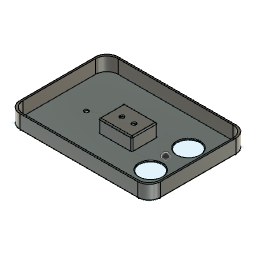
topo novo (Autodesk Fusion 360 design; units mm, degrees)
Autodesk Fusion 360 part; units mm, degrees
note: some values were not read from the file. Chosen so that the rebuilt part matches the saved one: which pieces of a blend or face edit are solid.
sketch "Esboço1" plane through (0, 0, 0) normal (0, 0, 1) x (1, 0, 0)
  line L0 (93, 65) -> (-93, 65)
  line L1 (-93, 65) -> (-93, -65)
  line L2 (-93, -65) -> (93, -65)
  line L3 (93, -65) -> (93, 65)
  line L4 (93, 65) -> (-93, -65) construction
  line L5 (-93, 65) -> (93, -65) construction
  dimension "d1" = 186
  dimension "d2" = 130
  constraint horizontal L0
  constraint perpendicular L0 L1
  constraint parallel L0 L2
  constraint parallel L1 L3
  constraint coincident L4 origin
  constraint coincident L5 origin
  measures "d1" distance of L1.end L2.end
  measures "d2" distance of L0.end L1.end
extrude "Extrusão1" add sketch "Esboço1" along normal blind 2
sketch "Esboço2" plane through (0, 0, 2) normal (0, 0, 1) x (-1, 0, 0)
  line L0 (-93, 65) -> (-93, -65)
  line L1 (-93, -65) -> (93, -65)
  line L2 (93, -65) -> (93, 65)
  line L3 (93, 65) -> (-93, 65)
  line L4 (-91, -63) -> (91, -63)
  line L5 (91, -63) -> (91, 63)
  line L6 (91, 63) -> (-91, 63)
  line L7 (-91, 63) -> (-91, -63)
  line L8 (-91, -63) -> (91, 63) construction
  line L9 (91, -63) -> (-91, 63) construction
  dimension "d5" = 182
  dimension "d6" = 126
  constraint horizontal L4
  constraint perpendicular L4 L5
  constraint parallel L4 L6
  constraint parallel L5 L7
  constraint coincident L8 origin
  constraint coincident L9 origin
  measures "d5" distance of L5.end L6.end
  measures "d6" distance of L4.end L5.end
extrude "Extrusão2" add sketch "Esboço2" along normal blind 38
extrude "Extrusão3" cut 1 faces at (-30.3333, 64.3333, 40) along direction (0, 0, -1) blind 20
sketch "Esboço3" plane through (0, 0, 2) normal (0, 0, 1) x (-1, 0, 0)
  line L0 (-91, -63) -> (91, -63)
  line L1 (91, -63) -> (91, 63)
  line L2 (91, 63) -> (-91, 63)
  line L3 (-91, 63) -> (-91, -63)
  point P0 (-50, 0)
  point P1 (-50, 0)
  constraint coincident P1 P0
sketch "Esboço4" plane through (0, 0, 2) normal (0, 0, 1) x (-1, 0, 0)
  line L0 (-23, -34.5) -> (-77, -34.5)
  line L1 (-77, -34.5) -> (-77, 34.5)
  line L2 (-23, 34.5) -> (-23, -34.5)
  line L3 (-23, -34.5) -> (-77, 34.5) construction
  line L4 (-77, -34.5) -> (-23, 34.5) construction
  line L5 (-21, -36.5) -> (-79, -36.5)
  line L6 (-79, -36.5) -> (-79, 36.5)
  line L7 (-21, 36.5) -> (-21, -36.5)
  line L8 (-21, -36.5) -> (-79, 36.5) construction
  line L9 (-79, -36.5) -> (-21, 36.5) construction
  line L10 (-23, 34.5) -> (-19, 38.5) construction
  line L11 (-19, 34.5) -> (-23, 38.5) construction
  line L12 (-77, 34.5) -> (-81, 38.5) construction
  line L13 (-81, 34.5) -> (-77, 38.5) construction
  line L14 (-77, 36.5) -> (-79, 36.5)
  line L15 (-77, 34.5) -> (-77, 36.5)
  line L16 (-21, 36.5) -> (-23, 36.5)
  line L17 (-23, 34.5) -> (-23, 36.5)
  line L18 (-77, 36.5) -> (-75, 36.5)
  line L19 (-75, 36.5) -> (-75, 34.5)
  line L20 (-75, 34.5) -> (-77, 34.5)
  line L21 (-77, 34.5) -> (-77, 36.5)
  line L22 (-23, 36.5) -> (-25, 36.5)
  line L23 (-25, 36.5) -> (-25, 34.5)
  line L24 (-25, 34.5) -> (-23, 34.5)
  line L25 (-23, 34.5) -> (-23, 36.5)
  point P0 (-50, 0)
  point P1 (-50, 0)
  point P2 (-21, 36.5)
  point P3 (-79, 36.5)
  dimension "d15" = 2
  dimension "d16" = 2
  constraint horizontal L0
  constraint perpendicular L0 L1
  constraint parallel L1 L2
  constraint coincident L3 P1
  constraint coincident L4 P1
  constraint horizontal L5
  constraint perpendicular L5 L6
  constraint parallel L6 L7
  constraint coincident L8 P1
  constraint coincident L9 P1
  constraint coincident P1 P0
  constraint coincident L10 P2
  constraint coincident L11 P2
  constraint coincident P2 L7.start
  constraint coincident L12 P3
  constraint coincident L13 P3
  constraint coincident P3 L6.end
  constraint perpendicular L6 L14
  constraint perpendicular L14 L15
  constraint perpendicular L16 L17
  constraint horizontal L18
  constraint vertical L19
  constraint horizontal L20
  constraint vertical L21
  constraint horizontal L22
  constraint vertical L23
  constraint horizontal L24
  constraint vertical L25
  measures "d15" distance of L14.start L18.end
  measures "d16" distance of L16.end L22.end
extrude "Extrusão4" add sketch "Esboço4" along normal blind 18 contours L0 L1 L2 L5 L6 L7 L14 L15 L16 L17 L21 L25
sketch "Esboço5" plane through (0, 0, 2) normal (0, 0, 1) x (-1, 0, 0)
  line L0 (-23, 36.5) -> (-25, 36.5)
  line L1 (-25, 36.5) -> (-25, 34.5)
  line L2 (-25, 34.5) -> (-23, 34.5)
  line L3 (-23, 34.5) -> (-23, 36.5)
  line L4 (-77, 34.5) -> (-75, 34.5)
  line L5 (-75, 34.5) -> (-75, 36.5)
  line L6 (-75, 36.5) -> (-77, 36.5)
  line L7 (-77, 36.5) -> (-77, 34.5)
  constraint horizontal L0
  constraint vertical L1
  constraint horizontal L2
  constraint vertical L3
  constraint horizontal L4
  constraint vertical L5
  constraint horizontal L6
  constraint vertical L7
extrude "Extrusão5" add sketch "Esboço5" along normal blind 18
extrude "Extrusão6" cut 1 faces at (75, -35.1667, 14) along direction (1, 0, 0) blind 1
extrude "Extrusão7" cut 1 faces at (78.3333, 11.5, 20) along direction (0, 0, -1) blind 10
fillet "Arredondamento1" radius 1 12 edges at (77.5, -36.5, 10) (79, 0, 10) (77, 0, 10) (76.5, -34.5, 10) (76, -35.5, 10) (21, 0, 10) (23, -36.5, 10) (25, -35.5, 10) (24, -34.5, 10) (23, 0, 10) (50, 36.5, 10) (50, 34.5, 10)
fillet "Arredondamento2" radius 15 8 edges at (-91, -63, 11) (-93, -65, 10) (93, -65, 10) (91, -63, 11) (93, 65, 10) (91, 63, 11) (-91, 63, 11) (-93, 65, 10)
delete_face "DeleteFace1" 1 faces at (23, -11.5, 4.3334)
fillet "Arredondamento3" radius 2 8 edges at (-93, 0, 0) (-88.6066, -60.6066, 0) (0, -65, 0) (88.6066, -60.6066, 0) (93, 0, 0) (88.6066, 60.6066, 0) (0, 65, 0) (-88.6066, 60.6066, 0)
sketch "Esboço6" plane through (0, 0, 0) normal (0, 0, -1) x (1, 0, 0)
  line L0 (-91, 50) -> (-91, -50)
  arc A0 (-91, -50) -> (-78, -63) centre (-78, -50) ccw
  line L1 (-78, -63) -> (78, -63)
  arc A1 (78, -63) -> (91, -50) centre (78, -50) ccw
  line L2 (91, -50) -> (91, 50)
  arc A2 (91, 50) -> (78, 63) centre (78, 50) ccw
  line L3 (78, 63) -> (-78, 63)
  arc A3 (-78, 63) -> (-91, 50) centre (-78, 50) ccw
  circle A4 centre (55, -25) radius 15
  circle A5 centre (55, 25) radius 15
  dimension "d39" = 30
  dimension "d41" = 30
  measures "d39" diameter of A4
  measures "d41" diameter of A5
extrude "Extrusão8" cut sketch "Esboço6" against normal blind 3 contours A4 | A5
sketch "Esboço7" plane through (0, 0, 2) normal (0, 0, 1) x (-1, 0, 0)
  line L0 (20, 15) -> (-20, 15)
  line L1 (-20, 15) -> (-20, -15)
  line L2 (-20, -15) -> (20, -15)
  line L3 (20, -15) -> (20, 15)
  line L4 (20, 15) -> (-20, -15) construction
  line L5 (-20, 15) -> (20, -15) construction
  line L6 (22, 17) -> (-22, 17)
  line L7 (-22, 17) -> (-22, -17)
  line L8 (-22, -17) -> (22, -17)
  line L9 (22, -17) -> (22, 17)
  line L10 (22, 17) -> (-22, -17) construction
  line L11 (-22, 17) -> (22, -17) construction
  dimension "d44" = 40
  dimension "d45" = 30
  dimension "d46" = 44
  dimension "d47" = 34
  constraint horizontal L0
  constraint perpendicular L0 L1
  constraint parallel L0 L2
  constraint parallel L1 L3
  constraint coincident L4 origin
  constraint coincident L5 origin
  constraint horizontal L6
  constraint perpendicular L6 L7
  constraint parallel L6 L8
  constraint parallel L7 L9
  constraint coincident L10 origin
  constraint coincident L11 origin
  measures "d44" distance of L1.end L2.end
  measures "d45" distance of L0.end L1.end
  measures "d46" distance of L7.end L8.end
  measures "d47" distance of L6.end L7.end
extrude "Extrusão9" add sketch "Esboço7" along normal blind 17
sketch "Esboço8" plane through (0, 0, 2) normal (0, 0, 1) x (-1, 0, 0)
  line L0 (-20, -15) -> (20, -15)
  line L1 (20, -15) -> (20, 15)
  line L2 (20, 15) -> (-20, 15)
  line L3 (-20, 15) -> (-20, -15)
  line L4 (-20, -15) -> (20, 15) construction
  line L5 (20, -15) -> (-20, 15) construction
  constraint horizontal L0
  constraint perpendicular L0 L1
  constraint parallel L0 L2
  constraint parallel L1 L3
  constraint coincident L4 origin
  constraint coincident L5 origin
extrude "Extrusão10" cut sketch "Esboço8" against normal blind 2
sketch "Esboço9" plane through (0, 0, 19) normal (0, 0, 1) x (-1, 0, 0)
  line L0 (20, 15) -> (20, -15)
  line L1 (20, -15) -> (-20, -15)
  line L2 (-20, -15) -> (-20, 15)
  line L3 (-20, 15) -> (20, 15)
  line L4 (22, -17) -> (22, 17)
  line L5 (22, 17) -> (-22, 17)
  line L6 (-22, 17) -> (-22, -17)
  line L7 (-22, -17) -> (22, -17)
  line L8 (22, 17) -> (-22, 17)
  line L9 (-22, 17) -> (-22, -17)
  line L10 (-22, -17) -> (22, -17)
  line L11 (22, -17) -> (22, 17)
  line L12 (22, 17) -> (-22, -17) construction
  line L13 (-22, 17) -> (22, -17) construction
  constraint horizontal L8
  constraint perpendicular L8 L9
  constraint parallel L8 L10
  constraint parallel L9 L11
  constraint coincident L12 origin
  constraint coincident L13 origin
  constraint coincident L4.end L5.start
extrude "Extrusão11" add sketch "Esboço9" against normal blind 2 contours L0 L1 L2 L3
fillet "Arredondamento4" radius 4 8 edges at (-20, 15, 8.5) (20, 15, 8.5) (20, -15, 8.5) (-20, -15, 8.5) (-20, 0, 0) (0, 15, 0) (20, 0, 0) (0, -15, 0)
fillet "Arredondamento5" radius 0.8 4 edges at (41.0151, 30.4242, 2) (41.0151, 19.5758, 0) (41.0151, -19.5758, 2) (41.0151, -30.4242, 0)
sketch "Esboço10" plane through (0, 0, 19) normal (0, 0, 1) x (-1, 0, 0)
  line L0 (22, -17) -> (22, 17)
  line L1 (22, 17) -> (-22, 17)
  line L2 (-22, 17) -> (-22, -17)
  line L3 (-22, -17) -> (22, -17)
  line L4 (22, 0) -> (20, 0)
  line L5 (20, 0) -> (8, 0)
  line L6 (-22, 0) -> (-20, 0)
  line L7 (-20, 0) -> (-8, 0)
  circle A0 centre (-8, 0) radius 2
  circle A1 centre (8, 0) radius 2
  dimension "d58" = 4
  dimension "d59" = 4
  constraint midpoint L0 L4.start
  constraint perpendicular L0 L4
  constraint perpendicular L0 L5
  constraint midpoint L2 L6.start
  constraint perpendicular L2 L6
  constraint perpendicular L2 L7
  constraint coincident L7.end A0.centre
  constraint coincident L5.end A1.centre
  measures "d58" diameter of A0
  measures "d59" diameter of A1
extrude "Extrusão12" cut sketch "Esboço10" against normal blind 2 contours A0 | A1
fillet "Arredondamento6" radius 0.8 4 edges at (-6.1353, 0.7232, 17) (-6.1353, -0.7232, 19) (9.8647, 0.7232, 17) (9.8647, -0.7232, 19)
fillet "Arredondamento7" radius 1.5 8 edges at (-22, 17, 10.5) (22, 17, 10.5) (0, 17, 19) (-22, 0, 19) (-22, -17, 10.5) (0, -17, 19) (22, -17, 10.5) (22, 0, 19)
sketch "Esboço11" plane through (0, 0, 0) normal (0, 0, -1) x (1, 0, 0)
  circle A0 centre (55, -25) radius 15.8
  line L0 (-91, 50) -> (-91, -50)
  arc A1 (-91, -50) -> (-78, -63) centre (-78, -50) ccw
  line L1 (-78, -63) -> (78, -63)
  arc A2 (78, -63) -> (91, -50) centre (78, -50) ccw
  line L2 (91, -50) -> (91, 50)
  arc A3 (91, 50) -> (78, 63) centre (78, 50) ccw
  line L3 (78, 63) -> (-78, 63)
  arc A4 (-78, 63) -> (-91, 50) centre (-78, 50) ccw
  arc A5 (-24, -11) -> (-16, -19) centre (-16, -11) ccw
  line L4 (-24, -11) -> (-24, 11)
  arc A6 (-16, 19) -> (-24, 11) centre (-16, 11) ccw
  line L5 (-16, 19) -> (16, 19)
  arc A7 (24, 11) -> (16, 19) centre (16, 11) ccw
  line L6 (24, 11) -> (24, -11)
  arc A8 (16, -19) -> (24, -11) centre (16, -11) ccw
  line L7 (16, -19) -> (-16, -19)
  circle A9 centre (55, 25) radius 15.8
  line L8 (-20, 0) -> (-50, 0)
  circle A10 centre (-55, 0) radius 2
  dimension "d66" = 4
  constraint perpendicular L4 L8
  measures "d66" diameter of A10
extrude "Extrusão13" cut sketch "Esboço11" against normal blind 2 contours A10
fillet "Arredondamento8" radius 0.8 2 edges at (-56.8647, 0.7232, 2) (-56.8647, -0.7232, 0)
sketch "Esboço12" plane through (0, 0, 2) normal (0, 0, 1) x (-1, 0, 0)
sketch "Esboço13" plane through (0, 0, 0) normal (0, 0, -1) x (1, 0, 0)
  circle A0 centre (55, 25) radius 15.8
  arc A1 (-24, -11) -> (-16, -19) centre (-16, -11) ccw
  line L0 (-24, -11) -> (-24, 11)
  arc A2 (-16, 19) -> (-24, 11) centre (-16, 11) ccw
  line L1 (-16, 19) -> (16, 19)
  arc A3 (24, 11) -> (16, 19) centre (16, 11) ccw
  line L2 (24, 11) -> (24, -11)
  arc A4 (16, -19) -> (24, -11) centre (16, -11) ccw
  line L3 (16, -19) -> (-16, -19)
  line L4 (-91, 50) -> (-91, -50)
  arc A5 (-91, -50) -> (-78, -63) centre (-78, -50) ccw
  line L5 (-78, -63) -> (78, -63)
  arc A6 (78, -63) -> (91, -50) centre (78, -50) ccw
  line L6 (91, -50) -> (91, 50)
  arc A7 (91, 50) -> (78, 63) centre (78, 50) ccw
  line L7 (78, 63) -> (-78, 63)
  arc A8 (-78, 63) -> (-91, 50) centre (-78, 50) ccw
  circle A9 centre (55, -25) radius 15.8
  circle A10 centre (-55, 0) radius 2.8
